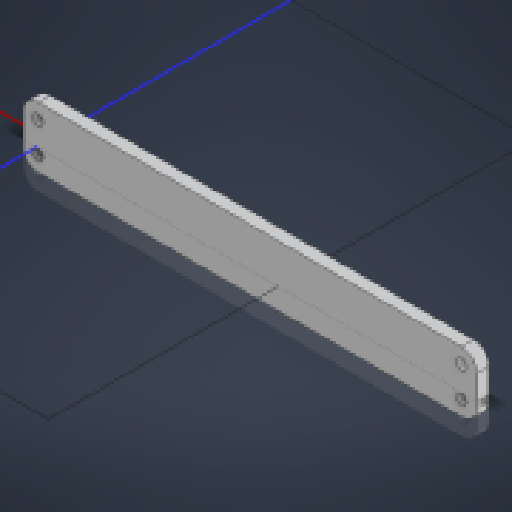
# Autodesk Inventor part: intakebrace
Saved by Autodesk Inventor 2025.2 (Build 292293000, 293)
## iProperties
Created: 2025-12-10
Part Number: intakebrace
Material: Generic
Document SubType Name: Modeling
Designer: cloudy
Density: 1 g/cm^3
Appearance: Default
Author: cloudy
Autodesk Inventor part; units mm, degrees
ref_plane "YZ Plane" through (0, 0, 0) normal (1, 0, 0) x (0, 1, 0)
ref_plane "XZ Plane" through (0, 0, 0) normal (0, 1, 0) x (-1, 0, 0)
ref_plane "XY Plane" through (0, 0, 0) normal (0, 0, 1) x (1, 0, 0)
sketch "Sketch1" plane through (0, 0, 0) normal (0, 0, 1) x (1, 0, 0)
  circle A0 centre (0.7751, -6.35) radius 2.1844 projected
  circle A1 centre (0.7751, 6.35) radius 2.1844 projected
  circle A2 centre (178.5751, 6.35) radius 2.1844 projected
  circle A3 centre (178.5751, -6.35) radius 2.1844 projected
  line L0 (178.5751, -12.7) -> (0.7751, -12.7)
  line L1 (-5.5749, -6.35) -> (-5.5749, 6.35)
  line L2 (0.7751, 12.7) -> (178.5751, 12.7)
  line L3 (184.9251, 6.35) -> (184.9251, -6.35)
  line L4 (184.9251, -12.7) -> (-5.5749, 12.7) construction
  line L5 (-5.5749, -12.7) -> (184.9251, 12.7) construction
  arc A4 (178.5751, -12.7) -> (184.9251, -6.35) centre (178.5751, -6.35) ccw
  arc A5 (184.9251, 6.35) -> (178.5751, 12.7) centre (178.5751, 6.35) ccw
  arc A6 (0.7751, 12.7) -> (-5.5749, 6.35) centre (0.7751, 6.35) ccw
  arc A7 (-5.5749, -6.35) -> (0.7751, -12.7) centre (0.7751, -6.35) ccw
  point P0 (0, 0)
  point P1 (89.6751, 0)
  dimension "d0" = 190.5
  dimension "d1" = 6.35
  dimension "d2" = 6.35
  dimension "d3" = 6.35
  dimension "d4" = 6.35
  constraints: 12 end point, 8 point on circle, 8 point on line, 8 tangent, 4 centre point, 3 equal radius, 2 midpoint, 2 parallel, 1 horizontal, 1 perpendicular
  measures "d0" distance of L4.end L5.end
  measures "d1" distance from line of L1 A1.centre
  measures "d2" distance from line of L2 A2.centre
  measures "d3" distance from line of A3.centre L0
  measures "d4" radius of A4
extrude "Extrusion1" add sketch "Sketch1" along normal blind 5.08
body "Solid1"
